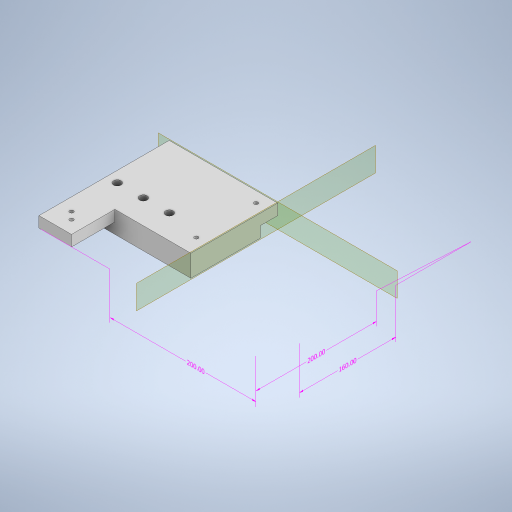
# Autodesk Inventor part: base_back_3
Saved by Autodesk Inventor 2023 (Build 270158000, 158)
## iProperties
Created: 2022-11-29
Part Number: base_back_3
Material: Genérico
Document SubType Name: Modeling
Designer: inigo
Density: 1 g/cm^3
Appearance: Valor por defecto
Author: inigo
Autodesk Inventor part; units mm, degrees
ref_plane "YZ Plane" through (0, 0, 0) normal (1, 0, 0) x (0, 1, 0)
ref_plane "XZ Plane" through (0, 0, 0) normal (0, 1, 0) x (-1, 0, 0)
ref_plane "XY Plane" through (0, 0, 0) normal (0, 0, 1) x (1, 0, 0)
sketch "Boceto1" plane through (0, 0, 0) normal (0, 1, 0) x (-1, 0, 0)
  line L0 (100, 80) -> (-100, 80)
  line L1 (-100, 80) -> (-100, -80)
  line L2 (-100, -80) -> (100, -80)
  line L3 (100, -80) -> (100, 80)
  line L4 (100, 80) -> (-100, -80) construction
  line L5 (-100, 80) -> (100, -80) construction
  point P0 (0, 0)
  dimension "d0" = 200
  dimension "d1" = 160
  constraints: 12 end point, 2 midpoint, 2 parallel, 1 horizontal, 1 perpendicular
  measures "d0" distance of L2.end L1.end
  measures "d1" distance of L1.end L0.end
extrude "Extrusión1" add sketch "Boceto1" along normal blind 20
sketch "Boceto2" plane through (0, 20, 0) normal (0, 1, 0) x (1, 0, 0)
  circle A0 centre (-90, -57.83) radius 3.5
  line L0 (-100, -65.43) -> (-32, -65.43)
  line L1 (-32, -65.43) -> (-32, 14.57)
  line L2 (-32, 14.57) -> (-100, 14.57)
  line L3 (-100, 14.57) -> (-100, -65.43)
  line L4 (-66, -65.43) -> (-66, -8.508)
  circle A1 centre (-66, -57.83) radius 3.5
  circle A2 centre (-42, -57.83) radius 3.5
  line L5 (-32, -25.43) -> (-48.2072, -25.43)
  circle A3 centre (-42, 6.97) radius 3.5
  circle A4 centre (-66, 6.97) radius 3.5
  circle A5 centre (-90, 6.97) radius 3.5
  circle A6 centre (-60, 55) radius 5
  line L6 (-100, 80) -> (-100, -80) projected
  line L7 (0, 0) -> (0, -20.5185)
  circle A7 centre (90, -57.83) radius 3.5
  circle A8 centre (66, -57.83) radius 3.5
  circle A9 centre (42, -57.83) radius 3.5
  line L8 (100, -65.43) -> (32, -65.43)
  line L9 (66, -65.43) -> (66, -8.508)
  line L10 (32, -25.43) -> (48.2072, -25.43)
  circle A10 centre (90, 6.97) radius 3.5
  line L11 (100, 14.57) -> (100, -65.43)
  circle A11 centre (66, 6.97) radius 3.5
  line L12 (32, 14.57) -> (100, 14.57)
  line L13 (32, -65.43) -> (32, 14.57)
  circle A12 centre (42, 6.97) radius 3.5
  circle A13 centre (60, 55) radius 5
  line L14 (100, 80) -> (100, -80)
  dimension "d4" = 7
  dimension "d5" = 68
  dimension "d6" = 80
  dimension "d7" = 7.6
  dimension "d8" = 10
  dimension "d9" = 7
  dimension "d10" = 24
  dimension "d11" = 10
  dimension "d16" = 0
  dimension "d19" = 40
  constraints: 28 end point, 21 symmetric about line, 14 centre point, 2 horizontal, 2 midpoint, 2 parallel, 2 point on line, 2 vertical, 1 perpendicular, 11 other
  measures "d4" diameter of A0
  measures "d5" distance of L3.start L2.start
  measures "d6" distance of L2.start L0.end
  measures "d7" distance from line of L0 A0.centre
  measures "d8" distance from line of L3 A0.centre
  measures "d9" diameter of A1
  measures "d10" distance of A4.centre A5.centre
  measures "d11" diameter of A6
  measures "d16" distance between parallel lines of L3 L6
  measures "d19" distance from line of L6 A6.centre
extrude "Extrusión2" cut sketch "Boceto2" against normal blind 20 contours A0 | A1 L4 | L4 A1 | A2 | A3 | A4 | A5 | A7 | A8 L9 | L9 A8 | A9 | A10 | A11 | A12
sketch "Boceto3" plane through (-100, 0, 80) normal (0, 0, 1) x (1, 0, 0)
  line L0 (0, 20) -> (30, 20)
  line L1 (30, 20) -> (30, 10)
  line L2 (30, 10) -> (0, 10)
  line L3 (0, 10) -> (0, 20)
  line L4 (100, 0) -> (100, 11.6249)
  line L5 (200, 20) -> (170, 20)
  line L6 (170, 20) -> (170, 10)
  line L7 (170, 10) -> (200, 10)
  line L8 (200, 10) -> (200, 20)
  dimension "d22" = 30
  dimension "d23" = 10
  constraints: 18 end point, 4 symmetric about line, 2 parallel, 1 horizontal, 1 perpendicular, 1 vertical
  measures "d22" distance of L1.end L2.end
  measures "d23" distance of L0.end L1.end
extrude "Extrusión3" add sketch "Boceto3" along normal blind 40
sketch "Boceto4" plane through (0, 20, 0) normal (0, 1, 0) x (1, 0, 0)
  line L0 (-60, 60) -> (-60, 50)
  line L1 (-70, 50) -> (-70, 60)
  line L2 (-60, 50) -> (-70, 60) construction
  line L3 (-70, 50) -> (-60, 60) construction
  line L4 (-60, 50) -> (-70, 50)
  circle A0 centre (-68.25, 51.75) radius 1.75
  line L5 (-70, 60) -> (-60, 60)
  circle A1 centre (-61.75, 58.25) radius 1.75
  line L6 (100, 80) -> (-100, 80) projected
  line L7 (0, 80) -> (0, 60)
  line L8 (60, 60) -> (60, 50)
  circle A2 centre (61.75, 58.25) radius 1.75
  line L9 (70, 60) -> (60, 60)
  line L10 (70, 50) -> (70, 60)
  line L11 (60, 50) -> (70, 60) construction
  line L12 (70, 50) -> (60, 60) construction
  line L13 (60, 50) -> (70, 50)
  circle A3 centre (68.25, 51.75) radius 1.75
  line L14 (-100, 80) -> (-100, -120) projected
  line L15 (100, 80) -> (100, -120) projected
  point P0 (0, 0)
  point P1 (-70.0286, 64.971)
  point P2 (-65, 50)
  point P3 (70.0286, 64.971)
  point P4 (65, 50)
  dimension "d26" = 1.75
  dimension "d27" = 8.25
  dimension "d28" = 20
  dimension "d29" = 10
  dimension "d30" = 10
  dimension "d31" = 1.75
  dimension "d32" = 1.75
  dimension "d33" = 1.75
  dimension "d58" = 30
  dimension "d59" = 30
  constraints: 22 end point, 8 symmetric about line, 4 centre point, 2 midpoint, 1 vertical, 8 other
  measures "d26" distance from line of L5 A1.centre
  measures "d27" distance from line of L5 A0.centre
  measures "d28" distance between parallel lines of L6 L5
  measures "d29" distance from line of point (-65, 50) L5
  measures "d30" length of L0
  measures "d31" distance from line of L4 A0.centre
  measures "d33" distance from line of L0 A1.centre
extrude "Extrusión4" cut sketch "Boceto4" against normal blind 40 contours A1 | A0 | A2 | A3
sketch "Boceto5" plane through (0, 20, 0) normal (0, 1, 0) x (1, 0, 0)
  line L0 (-100, -80) -> (-100, -120)
  line L1 (-70.0001, -120) -> (-70.0001, -80)
  line L2 (-55.1959, -79.9497) -> (-70.0001, -80)
  line L3 (-70.0001, -80) -> (-100, -80)
  line L4 (-100, -120) -> (-70.0001, -120)
  line L5 (-64.3507, -80) -> (-74.3507, -80)
  circle A0 centre (-81.75, -108.25) radius 1.75
  circle A1 centre (-88.25, -101.75) radius 1.75
  line L6 (-70.0001, -80) -> (70.0001, -80)
  line L7 (0, -80) -> (0, -101.75)
  circle A2 centre (81.75, -108.25) radius 1.75
  circle A3 centre (88.25, -101.75) radius 1.75
  line L8 (-70, -80) -> (70, -80) projected
  line L9 (-100, 80) -> (-100, -120) projected
  point P0 (0, 0)
  point P1 (-81.75, -101.75)
  point P2 (-63.4459, -118.25)
  point P3 (81.75, -101.75)
  dimension "d36" = 11.7499
  dimension "d37" = 40
  dimension "d38" = 29.9999
  dimension "d39" = 21.75
  dimension "d40" = 11.75
  dimension "d41" = 28.3003
  dimension "d42" = 11.7499
  dimension "d43" = 0
  dimension "d44" = 0
  constraints: 16 end point, 4 centre point, 3 symmetric about line, 1 midpoint, 1 vertical, 2 other
  measures "d36" distance from line of L1 point (-81.75, -101.75)
  measures "d37" distance between parallel lines of L4 L3
  measures "d38" distance between parallel lines of L0 L1
  measures "d39" vertical distance of L5.start A1.centre
  measures "d40" distance from line of L0 A1.centre
  measures "d41" vertical distance of L2.start A0.centre
  measures "d42" distance from line of L1 A0.centre
  measures "d43" distance between parallel lines of L8 L6
  measures "d44" distance between parallel lines of L9 L0
hole "Agujero1" at (-88.25, 20, 101.75) at (-81.75, 20, 108.25) at (81.75, 20, 108.25) at (88.25, 20, 101.75) direction (0, -1, 0) diameter 3.5 end through all
ref_plane "Plano de trabajo1" through (100, 0, 0) normal (0, 0, -1) x (-1, 0, 0)
ref_plane "Plano de trabajo2" through (0, 0, -80) normal (-1, 0, 0) x (0, 0, 1)
sketch "Boceto6" plane through (0, 0, 0) normal (0, -1, 0) x (1, 0, 0)
  circle A0 centre (10, -10) radius 1.75
  line L0 (6.803, 0) -> (14.6069, 0)
  line L1 (0, 0) -> (0, -4.8284)
  line L2 (0, 0) -> (20.0354, 0)
  circle A1 centre (10, 10) radius 1.75
  line L3 (0, 0) -> (0, 4.8284)
  circle A2 centre (-10, 10) radius 1.75
  circle A3 centre (-10, -10) radius 1.75
  dimension "d63" = 3.5
  dimension "d64" = 10
  dimension "d65" = 10
  constraints: 8 end point, 4 centre point, 4 symmetric about line, 2 horizontal, 1 vertical, 3 other
  measures "d63" diameter of A0
  measures "d64" distance from line of L1 A0.centre
  measures "d65" distance from line of L2 A0.centre
hole "Agujero2" at (10, 0, 10) at (-10, 0, 10) at (-10, 0, -10) at (10, 0, -10) direction (0, 1, 0) diameter 3.5 end through all
sketch "Boceto7" plane through (0, 0, 0) normal (0, -1, 0) x (1, 0, 0)
  line L0 (-16, 16) -> (16, 16)
  line L1 (16, 16) -> (16, -16)
  line L2 (16, -16) -> (-16, -16)
  line L3 (-16, -16) -> (-16, 16)
  line L4 (-16, 16) -> (16, -16) construction
  line L5 (16, 16) -> (-16, -16) construction
  point P0 (0, 0)
  point P1 (0, 0)
  point P2 (0, 0)
  dimension "d73" = 32
  dimension "d74" = 32
  constraints: 12 end point, 2 midpoint, 2 parallel, 1 horizontal, 1 perpendicular
  measures "d73" distance of L1.end L2.end
  measures "d74" distance of L0.end L1.end
extrude "Extrusión5" cut sketch "Boceto7" against normal blind 10
sketch "Boceto8" plane through (0, 20, 0) normal (0, 1, 0) x (1, 0, 0)
  line L0 (-15, -60) -> (15, -60)
  circle A0 centre (10, -65) radius 1.75
  line L1 (-10, -65) -> (10, -65)
  line L2 (15, -60) -> (15, -70)
  circle A1 centre (-10, -65) radius 1.75
  line L3 (-15, -70) -> (15, -60) construction
  line L4 (-15, -60) -> (15, -70) construction
  line L5 (-15, -70) -> (-15, -60)
  line L6 (15, -70) -> (-15, -70)
  point P0 (0, 0)
  point P1 (0, -69.1269)
  point P2 (-15, -67.1661)
  point P3 (0, -69.1269)
  point P4 (15, -65)
  dimension "d77" = 10
  dimension "d78" = 30
  dimension "d79" = 5
  dimension "d80" = 5
  dimension "d81" = 5
  dimension "d82" = 5
  constraints: 8 end point, 2 centre point, 1 midpoint, 9 other
  measures "d77" distance between parallel lines of L6 L0
  measures "d78" distance between parallel lines of L5 L2
  measures "d79" distance of point (15, -65) A0.centre
  measures "d80" distance from line of L0 A0.centre
  measures "d81" distance from line of L0 A1.centre
  measures "d82" distance from line of L5 A1.centre
hole "Agujero3" at (-10, 20, 65) at (10, 20, 65) direction (0, -1, 0) diameter 3.5 end through all
split "Dividir1" plane through (100, 0, 0) removes the side toward (0, 0, -1)
split "Dividir2" plane through (0, 0, -80) removes the side toward (1, 0, 0)
